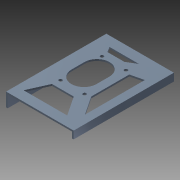
# Autodesk Inventor part: 15
Saved by Autodesk Inventor 2013 (Build 170138000, 138)
## iProperties
Created: 2013-12-28
Material: アルミニウム 6061
Document SubType Name: Modeling
Designer: andou
Density: 2.71 g/cm^3
Mass: 21.6993 g
Surface Area: 118.118 cm^2
Volume: 8.00713 cm^3
Part Number: 15
Author: andou
Title: Right_Sole
Autodesk Inventor part; units mm, degrees
ref_plane "YZ Plane" through (0, 0, 0) normal (1, 0, 0) x (0, 1, 0)
ref_plane "XZ Plane" through (0, 0, 0) normal (0, 1, 0) x (-1, 0, 0)
ref_plane "XY Plane" through (0, 0, 0) normal (0, 0, 1) x (1, 0, 0)
sketch "スケッチ1" plane through (0, 0, 0) normal (0, 0, 1) x (1, 0, 0)
  line L0 (-31, 46) -> (31, 46)
  line L1 (31, 46) -> (31, -46)
  line L2 (31, -46) -> (-31, -46)
  line L3 (-31, -46) -> (-31, 46)
  point P0 (0, 0)
  dimension "d0" = 92
  dimension "d1" = 46
  dimension "d2" = 62
  dimension "d3" = 31
  constraints: 8 end point, 2 parallel, 1 horizontal, 1 perpendicular
  measures "d0" distance of L2.end L0.start
  measures "d1" distance from line of L0 point (0, 0)
  measures "d2" distance of L1.end L2.end
  measures "d3" distance from line of L3 point (0, 0)
extrude "押し出し1" add sketch "スケッチ1" along normal blind 1.5
sketch "スケッチ3" plane through (0, 0, 0) normal (0, 0, -1) x (-1, 0, 0)
  circle A0 centre (-7, 26) radius 1.5
  circle A1 centre (15, 26) radius 1.5
  circle A2 centre (-7, -12) radius 1.5
  circle A3 centre (15, -12) radius 1.5
  line L0 (31, 46) -> (-31, 46) projected
  line L1 (31, -46) -> (31, 46) projected
  point P0 (0, 0)
  dimension "d10" = 3
  dimension "d11" = 22
  dimension "d12" = 22
  dimension "d15" = 38
  dimension "d16" = 38
  dimension "d35" = 20
  dimension "d36" = 20
  dimension "d44" = 16
  dimension "d45" = 16
  constraints: 4 centre point, 3 equal radius
  measures "d10" diameter of A0
  measures "d11" distance of A1.centre A0.centre
  measures "d12" distance of A3.centre A2.centre
  measures "d15" distance of A1.centre A3.centre
  measures "d16" distance of A2.centre A0.centre
  measures "d35" distance from line of L0 A0.centre
  measures "d36" distance from line of L0 A1.centre
  measures "d44" distance from line of L1 A1.centre
  measures "d45" distance from line of L1 A3.centre
hole "穴1" at (-15, -12, 0) at (-15, 26, 0) at (7, 26, 0) at (7, -12, 0) direction (0, 0, 1) diameter 3 end through all
sketch "スケッチ4" plane through (0, 0, 1.5) normal (0, 0, 1) x (1, 0, 0)
  line L0 (-31, -46) -> (-31, 46) projected
  line L1 (31, -46) -> (-31, -46) projected
  line L2 (-31, 46) -> (-29.5, 46)
  line L3 (-29.5, 46) -> (-29.5, -46)
  line L4 (-29.5, -46) -> (-31, -46)
  line L5 (-31, -46) -> (-31, 46)
  line L6 (31, 46) -> (29.5, 46)
  line L7 (29.5, 46) -> (29.5, -46)
  line L8 (29.5, -46) -> (31, -46)
  line L9 (31, -46) -> (31, 46)
  point P0 (0, 0)
  dimension "d37" = 59
  dimension "d39" = 1.5
  constraints: 16 end point, 4 parallel, 2 horizontal, 2 perpendicular, 2 point on line
  measures "d37" distance between parallel lines of L7 L3
  measures "d39" distance between parallel lines of L0 L3
extrude "押し出し3" add sketch "スケッチ4" against normal blind 12.5
sketch "スケッチ6" plane through (31, -46, 0) normal (1, 0, 0) x (0, 0, 1)
  line L0 (1.5, 0) -> (-11, 0) projected
  line L1 (-11, -92) -> (-5.5, -92)
  line L2 (-5.5, -92) -> (-5.5, 0)
  line L3 (-5.5, 0) -> (-11, 0)
  line L4 (-11, 0) -> (-11, -92)
  point P0 (0, 0)
  point P1 (0, -46)
  constraints: 8 end point, 2 parallel, 1 horizontal, 1 perpendicular, 1 point on line
extrude "押し出し5" cut sketch "スケッチ6" against normal blind 1.5
sketch "スケッチ7" plane through (0, 0, 1.5) normal (0, 0, 1) x (1, 0, 0)
  line L0 (4.5, 13.4115) -> (4.5, 1.4115)
  line L1 (-18.5, 1.4115) -> (-18.5, 13.4115)
  line L2 (-19, 36.9115) -> (8, 36.9115)
  line L3 (-0.3333, 31.9115) -> (-16, 31.9115)
  line L4 (-16, -18.9115) -> (4, -18.9115)
  line L5 (16, -36.9115) -> (-24, -36.9115)
  line L6 (-24, -36.9115) -> (-16, -18.9115)
  line L7 (16, -36.9115) -> (4, -18.9115)
  line L8 (-19, 36.9115) -> (-16, 31.9115)
  line L9 (8, 36.9115) -> (-0.3333, 31.9115)
  arc A0 (-18.5, 1.4115) -> (4.5, 1.4115) centre (-7, 1.4115) ccw
  arc A1 (4.5, 13.4115) -> (-18.5, 13.4115) centre (-7, 13.4115) ccw
  line L10 (31, -46) -> (31, 46) projected
  line L11 (12, -10.9115) -> (23.5, -28.1615)
  line L12 (23.5, -28.1615) -> (23.5, 26.8385)
  line L13 (23.5, 26.8385) -> (12, 24.0885)
  line L14 (12, -10.9115) -> (12, 24.0885)
  line L15 (29.5, 46) -> (29.5, -46) projected
  line L16 (-29.5, 46) -> (29.5, 46) projected
  point P0 (0, 0)
  dimension "d62" = 12
  dimension "d63" = 11.5
  dimension "d64" = 11.5
  dimension "d65" = 23
  dimension "d70" = 5
  dimension "d72" = 18
  dimension "d73" = 27
  dimension "d89" = 40
  dimension "d92" = 20
  dimension "d114" = 35
  dimension "d115" = 55
  dimension "d118" = 11.5
  dimension "d119" = 6
  dimension "d125" = 38
  dimension "d126" = 9.0885
  constraints: 28 end point, 6 parallel, 4 point on circle, 2 centre point, 2 horizontal, 1 perpendicular
  measures "d62" distance of A1.centre A0.centre
  measures "d63" radius of A0
  measures "d64" radius of A1
  measures "d65" distance between parallel lines of L0 L1
  measures "d70" distance between parallel lines of L3 L2
  measures "d72" distance between parallel lines of L4 L5
  measures "d73" distance of L2.start L2.end
  measures "d89" distance of L5.start L5.end
  measures "d92" distance of L4.start L4.end
  measures "d114" distance of L11.start L13.end
  measures "d115" distance of L11.end L12.end
  measures "d118" distance between parallel lines of L12 L14
  measures "d119" distance between parallel lines of L15 L12
  measures "d125" distance from line of L10 A1.centre
  measures "d126" distance between parallel lines of L16 L2
extrude "押し出し7" cut sketch "スケッチ7" against normal blind 1.5
